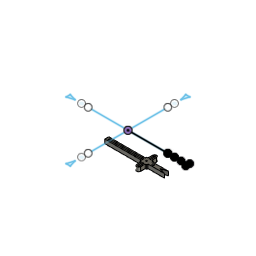
2023_01_30_FootCalibration For LaserCNCPlotter v1 (Autodesk Fusion 360 design; units mm, degrees)
Autodesk Fusion 360 part; units mm, degrees
note: some values were not read from the file. Set by a fixed rule: which face or edge a step refers to.
sketch "Esquisse2" plane through (0, 0, 0) normal (0, 0, 1) x (1, 0, 0)
  line L0 (45, 1.5165) -> (-0.0003, 1.5085)
  line L1 (31.5, -6) -> (31.5, 6)
  line L2 (1.5, -0.5) -> (1.5, 0.5)
  line L3 (0.0003, -1.4915) -> (45, -1.4835)
  line L4 (-0.0003, 1.5085) -> (0.0003, -1.4915)
  line L5 (40, 0) -> (45, 1.5165)
  line L6 (40, 0) -> (45, 1.5165)
  line L7 (45, 1.5165) -> (-0.0003, 1.5085)
  line L8 (45, -1.4835) -> (40, 0)
  line L9 (1.5, -0.5) -> (1.5, 0.5)
  arc A0 (31.5, 6) -> (28.5, 6) centre (30, 6) ccw
  line L10 (28.5, 6) -> (28.5, -6)
  circle A1 centre (35, 0) radius 0.75
  line L11 (30, 6) -> (30, -6)
  line L12 (1.5, 0.5) -> (28.5, 0.5)
  circle A2 centre (30, 0) radius 0.5
  line L13 (29.5, 6) -> (29.5, -6)
  line L14 (0.0003, -1.4915) -> (45, -1.4835)
  line L15 (1.5, 0.5) -> (28.5, 0.5)
  line L16 (28.5, -0.5) -> (1.5, -0.5)
  line L17 (28.5, -0.5) -> (1.5, -0.5)
  line L18 (45, -1.4835) -> (40, 0)
  line L19 (-0.0003, 1.5085) -> (0.0003, -1.4915)
  line L20 (30, 6) -> (30, -6)
  circle A3 centre (30, 0) radius 0.5
  arc A4 (29.5, -6) -> (30.5, -6) centre (30, -6) ccw
  arc A5 (28.5, -6) -> (31.5, -6) centre (30, -6) ccw
  arc A6 (30.5, 6) -> (29.5, 6) centre (30, 6) ccw
  line L21 (30.5, -6) -> (30.5, 6)
  line L22 (32.5, 2.5) -> (27.5, 2.5)
  line L23 (27.5, 2.5) -> (27.5, -2.5)
  line L24 (27.5, -2.5) -> (32.5, -2.5)
  line L25 (32.5, -2.5) -> (32.5, 2.5)
  line L26 (32.5, 2.5) -> (27.5, -2.5) construction
  line L27 (27.5, 2.5) -> (32.5, -2.5) construction
  line L28 (0, 6) -> (45, 6) construction
  line L29 (45, 6) -> (45, -2) construction
  point P0 (30, 0)
  dimension "d8" = 1.5
  constraint horizontal L22
  constraint perpendicular L22 L23
  constraint parallel L22 L24
  constraint parallel L23 L25
  constraint coincident L26 P0
  constraint coincident L27 P0
  constraint coincident P0 A2.centre
  constraint perpendicular L0 L4
  constraint perpendicular L4 L14
  constraint perpendicular L13 L28
  constraint perpendicular L28 L29
  constraint coincident L0.start L29
  constraint coincident L3.end L29
  constraint coincident L10 L12.end
  constraint coincident L10 L16.start
  measures "d8" diameter of A1
extrude "Extrusion1" add sketch "Esquisse2" along normal blind 3 contours L0 L3 L5 L6 L7 L8 L14 L18 L25 | L0 L1 L3 L7 L14 L25 | L0 L1 L7 L22 L25 | L0 L1 L3 L7 L14 L21 | L0 L1 L7 L21 L22 | L1 L3 L14 L24 L25 | L0 L7 L11 A2 L20 A3 L21 | L0 L7 L11 L20 L21 L22 | L1 L3 L14 L21 L24 | L1 A0 L10 L13 A6 L21 L22 | L0 L7 L11 A2 L13 L20 A3 | L0 L7 L11 L13 L20 L22 | L3 L11 A2 L14 L20 A3 L21 | L1 L10 L13 A4 A5 L21 L24 | L3 L11 L14 L20 L21 L24 | L0 L3 L7 L10 L13 L14 | L0 L7 L10 L13 L22 | L3 L11 A2 L13 L14 L20 A3 | L3 L11 L13 L14 L20 L24 | L0 L7 L10 L12 L15 L23 | L0 L7 L10 L22 L23 | L3 L10 L13 L14 L24 | L0 L2 L3 L4 L7 L9 L12 L14 L15 L16 L17 L19 L23 | L10 L12 L15 L16 L17 L23 | L3 L10 L14 L23 L24 | L3 L10 L14 L16 L17 L23 makes body 1
copy_body "Copier/Coller des corps1" bodies 1 makes body 2
move_body "Déplacer1" bodies 2 to x (1, 0, 0) y (0, 1, 0) z (0, 0, 1) at (0, -16, 0)
draft "Dépouille1" angle -20 neutral plane through (0, 0, 0) pull (0, 0, -1) 4 faces at (30.1635, -0.4725, 2) (29.8365, -0.4725, 2) (29.6381, 0.345, 2) (30.1179, 0.4859, 2) on bodies 1
sketch "Esquisse3" plane through (0, 0, 0) normal (0, 0, 1) x (1, 0, 0)
  line L0 (0, 0) -> (30, 0)
  circle A0 centre (30, 0) radius 0.05
  circle A1 centre (35, 0) radius 0.05
  circle A2 centre (30, 0) radius 0.5
  circle A3 centre (35, 0) radius 0.7616
  line L1 (40, 0) -> (45, 1.5165)
  line L2 (45, 1.5165) -> (45, -1.4835)
  line L3 (45, -1.4835) -> (40, 0)
  line L4 (30, 0) -> (35, 0) construction
  line L5 (35, 0) -> (40, 0) construction
  point P0 (30, 0)
  point P1 (35, 0)
  point P2 (40, 0)
  point P3 (45, 1.5165)
  point P4 (45, -1.4835)
  dimension "d9" = 30
  dimension "d10" = 0.1
  dimension "d11" = 0.1
  dimension "d12" = 5
  dimension "d13" = 5
  constraint coincident L0.start origin
  constraint coincident P0 L0.end
  constraint coincident P1 A1.centre
  constraint concentric A0 A2
  constraint coincident P2 L1.start
  constraint coincident P3 L1.end
  constraint coincident P4 L2.end
  measures "d9" distance of L0.start P0
  measures "d10" diameter of A0
  measures "d11" diameter of A1
  measures "d12" distance of P0 P1
  measures "d13" distance of P2 P1
sketch "Esquisse4" plane through (0, 0, 0) normal (0, 0, 1) x (1, 0, 0)
  line L0 (0, 0) -> (30, 0)
  line L1 (45, 1.5165) -> (45, -1.4835)
  line L2 (40, 0) -> (45, 1.5165)
  line L3 (45, -1.4835) -> (40, 0)
  circle A0 centre (35, 0) radius 0.7616
  line L4 (0, 0) -> (0, 30)
  line L5 (1.4835, 45) -> (0, 40)
  line L6 (-1.5165, 45) -> (1.4835, 45)
  line L7 (0, 40) -> (-1.5165, 45)
  circle A1 centre (0, 35) radius 0.7616
  line L8 (0, 0) -> (-30, 0)
  line L9 (-45, 1.4835) -> (-40, 0)
  line L10 (-45, -1.5165) -> (-45, 1.4835)
  line L11 (-40, 0) -> (-45, -1.5165)
  circle A2 centre (-35, 0) radius 0.7616
  line L12 (0, 0) -> (0, -30)
  line L13 (-1.4835, -45) -> (0, -40)
  line L14 (1.5165, -45) -> (-1.4835, -45)
  line L15 (0, -40) -> (1.5165, -45)
  circle A3 centre (0, -35) radius 0.7616
  circle A4 centre (30, 0) radius 0.05
  point P0 (0, 30)
  point P1 (-30, 0)
  point P2 (0, -30)
  dimension "d14" = 30
  dimension "d16" = 360
  dimension "d17" = 0.1
  dimension "d19" = 360
  constraint coincident L0.end A4.centre
  measures "d14" distance of L0.end L0.start
  measures "d17" diameter of A4
hidden bodies 1
named bodies: "FotCalibration Straigh Solid", "FotCalibration Straigh Solid (1)"
